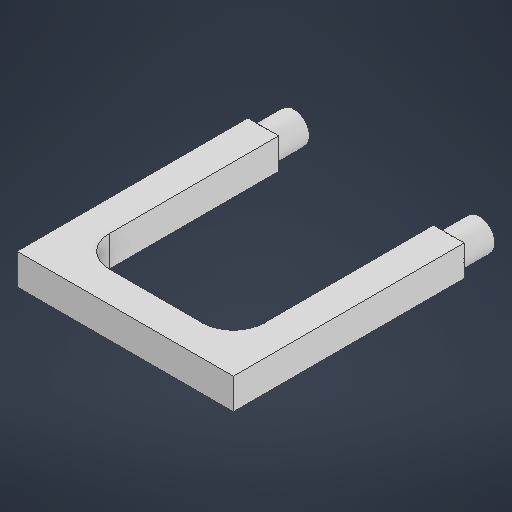
# Autodesk Inventor part: Trem_Pouso
Saved by Autodesk Inventor 2027 (Build 310192000, 192)
## iProperties
Created: 2026-07-11
Part Number: Trem_Pouso
Material: Genérico
Document SubType Name: Modeling
Designer: marcu
Density: 1 g/cm^3
Appearance: Padrão
Author: marcu
Autodesk Inventor part; units mm, degrees
ref_plane "YZ Plane" through (0, 0, 0) normal (1, 0, 0) x (0, 1, 0)
ref_plane "XZ Plane" through (0, 0, 0) normal (0, 1, 0) x (-1, 0, 0)
ref_plane "XY Plane" through (0, 0, 0) normal (0, 0, 1) x (1, 0, 0)
sketch "Esboço1" plane through (0, 0, 0) normal (0, 0, 1) x (1, 0, 0)
  circle A0 centre (0, 0) radius 1
  line L0 (0, 0) -> (12.0565, 0) construction
  circle A1 centre (12.0565, 0) radius 1
  dimension "d0" = 2
  dimension "d1" = 12.0565
  dimension "d2" = 2
  constraints: 2 centre point, 2 coincident, 2 end point, 1 horizontal
  measures "d0" diameter of A0
  measures "d1" distance of L0.start L0.end
  measures "d2" diameter of A1
extrude "Extrusão1" add sketch "Esboço1" along normal blind 2
sketch "Esboço2" plane through (0, 0, 2) normal (0, 0, 1) x (1, 0, 0)
  line L0 (-1, 1) -> (1, 1)
  line L1 (1, 1) -> (1, -1)
  line L2 (1, -1) -> (-1, -1)
  line L3 (-1, -1) -> (-1, 1)
  circle A0 centre (0, 0) radius 1 projected
  line L4 (-1, 1) -> (1, -1) construction
  line L5 (1, 1) -> (-1, -1) construction
  circle A1 centre (12.0565, 0) radius 1 projected
  line L6 (0, 0) -> (12.0565, 0) construction
  line L7 (11.0565, 1) -> (13.0565, 1)
  line L8 (13.0565, 1) -> (13.0565, -1)
  line L9 (13.0565, -1) -> (11.0565, -1)
  line L10 (11.0565, -1) -> (11.0565, 1)
  line L11 (11.0565, 1) -> (13.0565, -1) construction
  line L12 (13.0565, 1) -> (11.0565, -1) construction
  constraints: 26 end point, 4 midpoint, 4 parallel, 4 tangent, 3 horizontal, 2 perpendicular
extrude "Extrusão2" add sketch "Esboço2" along normal blind 15
sketch "Esboço3" plane through (0, 0, 17) normal (0, 0, 1) x (1, 0, 0)
  line L0 (1, 0) -> (1, 1) projected
  line L1 (12.0565, 1) -> (11.0565, 1) projected
  line L2 (1, 1) -> (11.0565, 1)
  line L3 (11.0565, 1) -> (11.0565, -1)
  line L4 (11.0565, -1) -> (1, -1)
  line L5 (1, -1) -> (1, 1)
  point P0 (0, 0)
  dimension "d7" = 2
  constraints: 8 end point, 2 parallel, 1 horizontal, 1 perpendicular
  measures "d7" distance between parallel lines of L1 L4
extrude "Extrusão3" add sketch "Esboço3" against normal blind 2
fillet "Arredondamento1" radius 2 2 edges at (11.0565, 0, 15) (1, 0, 15)
